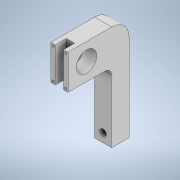
# Autodesk Inventor part: Ch7(5) Part 13 Column
Saved by Autodesk Inventor 2020 (Build 240168000, 168)
## iProperties
Created: 2021-03-08
Part Number: Ch7(5) Part 13 Column
Material: Generic
Document SubType Name: Modeling
Designer: austi
Density: 1 g/cm^3
Appearance: Default
Author: austi
Autodesk Inventor part; units mm, degrees
ref_plane "YZ Plane" through (0, 0, 0) normal (1, 0, 0) x (0, 1, 0)
ref_plane "XZ Plane" through (0, 0, 0) normal (0, 1, 0) x (-1, 0, 0)
ref_plane "XY Plane" through (0, 0, 0) normal (0, 0, 1) x (1, 0, 0)
sketch "Sketch1" plane through (0, 0, 0) normal (1, 0, 0) x (0, 1, 0)
  line L0 (0, -112.9926) -> (0, 18.8321) projected
  line L1 (-133.1321, 0) -> (87.5926, 0) projected
  line L2 (0, 0) -> (50.8, 0)
  line L3 (50.8, 0) -> (50.8, -63.5)
  line L4 (25.4, -88.9) -> (-101.6, -88.9)
  line L5 (-101.6, -88.9) -> (-101.6, -63.5)
  line L6 (-101.6, -63.5) -> (-9.652, -63.5)
  line L7 (0, 0) -> (0, -53.848)
  arc A0 (25.4, -88.9) -> (50.8, -63.5) centre (25.4, -63.5) ccw
  arc A1 (-9.652, -63.5) -> (0, -53.848) centre (-9.652, -53.848) ccw
  point P0 (50.8, -88.9)
  point P1 (0, -63.5)
  dimension "d0" = 50.8
  dimension "d1" = 88.9
  dimension "d2" = 152.4
  dimension "d3" = 25.4
  dimension "d4" = 25.4
  dimension "d5" = 9.652
  constraints: 12 end point, 6 point on line, 4 point on circle, 4 tangent, 3 perpendicular, 2 centre point, 1 collinear, 1 parallel
  measures "d0" distance of L2.start L2.end
  measures "d1" distance of L2.end point (50.8, -88.9)
  measures "d2" distance of point (50.8, -88.9) L4.end
  measures "d3" distance of L4.end L5.end
  measures "d4" radius of A0
  measures "d5" radius of A1
extrude "Extrusion1" add sketch "Sketch1" against normal blind 24.8285
sketch "Sketch6" plane through (0, -101.6, -88.9) normal (0, 0, -1) x (-1, 0, 0)
  circle A0 centre (12.4142, 12.7) radius 4.953
  line L0 (0, 0) -> (24.8285, 0) projected
  point P0 (0, 101.6)
  point P1 (12.4142, 0)
  dimension "d16" = 9.906
  dimension "d17" = 12.7
  constraints: 1 centre point, 1 midpoint, 1 vertical alignment
  measures "d16" diameter of A0
  measures "d17" vertical distance of L0.start A0.centre
extrude "Extrusion4" cut sketch "Sketch6" against normal through all
sketch "Sketch7" plane through (0, -101.6, -88.9) normal (0, 0, -1) x (-1, 0, 0)
  circle A0 centre (12.4142, 12.7) radius 7.1374
  circle A1 centre (12.4142, 12.7) radius 4.953 projected
  point P0 (0, 101.6)
  dimension "d20" = 14.2748
  constraints: 1 centre point, 1 concentric
  measures "d20" diameter of A0
extrude "Extrusion5" cut sketch "Sketch7" against normal blind 9.525
sketch "Sketch8" plane through (0, 0, 0) normal (0, 0, 1) x (1, 0, 0)
  line L0 (0, 0) -> (-24.8285, 0) projected
  line L1 (-6.35, 50.8) -> (-6.35, 0)
  line L2 (-18.4785, 50.8) -> (-18.4785, 0)
  line L3 (0, 25.4) -> (0, 50.8) projected
  line L4 (-6.35, 50.8) -> (0, 50.8)
  line L5 (0, 0) -> (0, -9.652) projected
  line L6 (0, 50.8) -> (0, 0)
  line L7 (0, 0) -> (-6.35, 0)
  line L8 (-24.8285, 50.8) -> (-18.4785, 50.8)
  line L9 (-24.8285, 0) -> (-18.4785, 0)
  line L10 (-24.8285, 0) -> (-24.8285, 50.8) projected
  line L11 (-18.4785, 50.8) -> (-6.35, 50.8)
  line L12 (0, 50.8) -> (-24.8285, 50.8) projected
  line L13 (-18.4785, 0) -> (-6.35, 0)
  line L14 (0, 0) -> (-24.8285, 0) projected
  dimension "d23" = 6.35
  dimension "d24" = 6.35
  constraints: 18 end point, 4 collinear, 2 perpendicular, 2 point on line, 1 horizontal, 1 vertical
  measures "d23" distance from line of L1 L3.end
  measures "d24" distance between parallel lines of L2 L10
extrude "Extrusion6" cut sketch "Sketch8" against normal blind 15.875 contours L0 L2 L11 L1
sketch "Sketch9" plane through (-24.8285, 0, 0) normal (0, 0, 1) x (1, 0, 0)
  line L0 (6.35, 50.8) -> (0, 50.8) projected
  line L1 (24.8285, 50.8) -> (18.4785, 50.8) projected
  line L2 (24.8285, 0) -> (18.4785, 0) projected
  line L3 (6.35, 0) -> (0, 0) projected
  point P0 (3.175, 47.625)
  point P1 (21.6535, 47.625)
  point P2 (21.6535, 3.175)
  point P3 (3.175, 3.175)
  point P4 (3.175, 50.8)
  point P5 (21.6535, 50.8)
  point P6 (21.6535, 0)
  dimension "d27" = 3.175
  dimension "d28" = 3.175
  constraints: 5 vertical alignment, 3 midpoint, 2 horizontal alignment
  measures "d27" distance from line of L0 point (3.175, 47.625)
  measures "d28" distance from line of L3 point (3.175, 3.175)
hole "Hole1" at (-21.6535, 47.625, 0) at (-3.175, 47.625, 0) at (-3.175, 3.175, 0) at (-21.6535, 3.175, 0) direction (0, 0, -1) diameter 3.302 depth 11.1252 tip angle 118 thread size "8-32 UNC" class "2B" standard "ANSI Unified Screw Threads"
sketch "Sketch10" plane through (0, 0, 0) normal (1, 0, 0) x (0, 0, -1)
  line L0 (0, 50.8) -> (0, 0) projected
  point P0 (26.9748, 25.4)
  point P1 (0, 25.4)
  dimension "d36" = 26.9748
  constraints: 1 horizontal alignment, 1 midpoint
  measures "d36" horizontal distance of point (26.975, 25.4) L0.end
hole "Hole2" at (0, 25.4, -26.9748) direction (-1, 0, 0) diameter 12.7 end through all counterbore diameter 29.718 counterbore depth 19.7104
body "Solid1"
